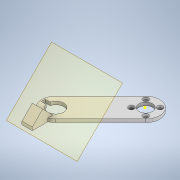
# Autodesk Inventor part: Pièce_moteur_maintient_test_6
Saved by Autodesk Inventor 2020.1 (Build 241239000, 239)
## iProperties
Created: 2019-07-26
Part Number: Pièce_moteur_maintient_test_6
Material: Générique
Document SubType Name: Modeling
Designer: marlo
Density: 1 g/cm^3
Appearance: Par défaut
Author: marlo
Autodesk Inventor part; units mm, degrees
ref_plane "YZ Plane" through (0, 0, 0) normal (1, 0, 0) x (0, 1, 0)
ref_plane "XZ Plane" through (0, 0, 0) normal (0, 1, 0) x (-1, 0, 0)
ref_plane "XY Plane" through (0, 0, 0) normal (0, 0, 1) x (1, 0, 0)
sketch "Esquisse3" plane through (0, 0, 0) normal (0, 1, 0) x (-1, 0, 0)
  line L0 (-7.087, 5.913) -> (5.913, 5.913) construction
  line L1 (5.913, 5.913) -> (5.913, -7.087) construction
  line L2 (5.913, -7.087) -> (-7.087, -7.087) construction
  line L3 (-7.087, -7.087) -> (-7.087, 5.913) construction
  line L4 (-7.087, 5.913) -> (5.913, -7.087) construction
  line L5 (5.913, 5.913) -> (-7.087, -7.087) construction
  line L6 (-12.087, 10.913) -> (10.913, 10.913) construction
  line L7 (10.913, 10.913) -> (10.913, -12.087) construction
  line L8 (10.913, -12.087) -> (-12.087, -12.087) construction
  line L9 (-12.087, -12.087) -> (-12.087, 10.913) construction
  line L10 (-12.087, 10.913) -> (10.913, -12.087) construction
  line L11 (10.913, 10.913) -> (-12.087, -12.087) construction
  line L12 (-7.087, 5.913) -> (-12.087, 5.913) construction
  line L13 (-12.087, 5.913) -> (-12.087, 10.913) construction
  line L14 (-12.087, 10.913) -> (-7.087, 10.913) construction
  line L15 (-7.087, 10.913) -> (-7.087, 5.913) construction
  line L16 (-7.087, -7.087) -> (-12.087, -7.087) construction
  line L17 (-12.087, -7.087) -> (-12.087, -12.087) construction
  line L18 (-12.087, -12.087) -> (-7.087, -12.087) construction
  line L19 (-7.087, -12.087) -> (-7.087, -7.087) construction
  line L20 (5.913, -7.087) -> (10.913, -7.087) construction
  line L21 (10.913, -7.087) -> (10.913, -12.087) construction
  line L22 (10.913, -12.087) -> (5.913, -12.087) construction
  line L23 (5.913, -12.087) -> (5.913, -7.087) construction
  line L24 (10.913, 10.913) -> (5.913, 10.913) construction
  line L25 (5.913, 10.913) -> (5.913, 5.913) construction
  line L26 (5.913, 5.913) -> (10.913, 5.913) construction
  line L27 (10.913, 5.913) -> (10.913, 10.913) construction
  circle A0 centre (8.413, 8.413) radius 2.5
  circle A1 centre (8.413, -9.587) radius 2.5
  circle A2 centre (-9.587, -9.587) radius 2.5
  circle A3 centre (-9.587, 8.413) radius 2.5
  circle A4 centre (-0.587, -0.587) radius 17.5
  circle A5 centre (-0.587, -0.587) radius 8.5
  circle A6 centre (55.9815, 55.9815) radius 17.5
  circle A7 centre (55.9815, 55.9815) radius 10
  line L28 (57.4815, 65.8684) -> (54.4815, 65.8684)
  line L29 (54.4815, 65.8684) -> (54.4815, 86.8684)
  line L30 (54.4815, 86.8684) -> (57.4815, 86.8684)
  line L31 (57.4815, 86.8684) -> (57.4815, 65.8684)
  line L32 (49.4815, 91.8684) -> (49.4815, 60.8684)
  line L33 (49.4815, 60.8684) -> (62.4815, 60.8684)
  line L34 (62.4815, 60.8684) -> (62.4815, 91.8684)
  line L35 (62.4815, 91.8684) -> (49.4815, 91.8684)
  line L36 (71.664, 53.4815) -> (65.664, 53.4815)
  line L37 (65.664, 53.4815) -> (65.664, 58.4815)
  line L38 (65.664, 58.4815) -> (71.664, 58.4815)
  line L39 (71.664, 58.4815) -> (71.664, 53.4815)
  line L40 (11.7873, -12.9614) -> (-12.9614, 11.7873) construction
  line L41 (11.7873, -12.9614) -> (68.3559, 43.6071)
  line L42 (-12.9614, 11.7873) -> (43.6071, 68.3559)
  line L43 (-12.9614, -12.9614) -> (68.3559, 68.3559) construction
  point P0 (-0.587, -0.587)
  point P1 (8.413, 8.413)
  point P2 (73.4815, 55.9815)
  point P3 (17.4356, 66.5)
  point P4 (62.4815, 72.2296)
  point P5 (49.4815, 72.2296)
  point P6 (57.4815, 73.4171)
  point P7 (54.4815, 73.4171)
  point P8 (49.4815, 63.5808)
  point P9 (62.4815, 63.5808)
  dimension "d1" = 13
  dimension "d2" = 13
  dimension "d3" = 5
  dimension "d4" = 35
  dimension "d9" = 9
  dimension "d31" = 35
  dimension "d32" = 20
  dimension "d33" = 3
  dimension "d34" = 21
  dimension "d36" = 5
  dimension "d37" = 5
  dimension "d51" = 6
  dimension "d56" = 115
  constraints: 88 end point, 20 parallel, 12 tangent, 11 point on circle, 9 perpendicular, 8 centre point, 8 horizontal, 6 coincident, 4 collinear, 2 midpoint, 2 point on line, 3 other
  measures "d1" distance of L0.end L1.end
  measures "d2" distance of L0.start L0.end
  measures "d3" distance between parallel lines of L2 L8
  measures "d4" diameter of A4
  measures "d9" radial gap between concentric circles of A4 A5
  measures "d31" diameter of A6
  measures "d32" diameter of A7
  measures "d33" distance of L29.end L30.end
  measures "d34" distance of L30.end L28.start
  measures "d36" distance between parallel lines of L29 L32
  measures "d37" distance of L38.end L36.start
  measures "d51" distance of L36.start L36.end
  measures "d56" distance of L43.start L43.end
extrude "Extrusion1" add sketch "Esquisse3" along normal blind 4 contours A4 | A4 L42 A6 L41 | A6 L32 A7 L36 L39 L38 L34 | L32 L35 L34 A6 L31 L30 L29 | A6 L29 A7 L32 | L34 A7 L31 A6
chamfer "Chanfrein5" distance 1 distance2 2 1 edges at (12.087, 4, -9.587) measured on face at (12.587, 4, -9.587)
chamfer "Chanfrein6" distance 1 distance2 2 1 edges at (-5.913, 4, -9.587) measured on face at (-5.413, 4, -9.587)
chamfer "Chanfrein7" distance 1 distance2 2 1 edges at (-5.913, 4, 8.413) measured on face at (-5.413, 4, 8.413)
chamfer "Chanfrein8" distance 1 distance2 2 1 edges at (12.087, 4, 8.413) measured on face at (12.587, 4, 8.413)
ref_plane "Plan de construction1" through (-62.4815, 4, 91.8684) normal (0, 0.7071068, 0.7071068) x (1, 0, 0)
sketch "Esquisse8" plane through (-62.4815, 4, 91.8684) normal (0, 0.7071068, 0.7071068) x (1, 0, 0)
  line L0 (0, 11.0583) -> (0, -2.8284) projected
  line L1 (0, 0) -> (13, 0)
  line L2 (13, 0) -> (13, 18.3465)
  line L3 (13, 18.3465) -> (0, 18.3465)
  line L4 (0, 18.3465) -> (0, 0)
  line L5 (8, 3.5355) -> (5, 3.5355) projected
  line L6 (8, 3.5355) -> (5, 3.5355)
  line L7 (5, 3.5355) -> (5, 18.3465)
  line L8 (5, 18.3465) -> (8, 18.3465)
  line L9 (8, 18.3465) -> (8, 3.5355)
  point P0 (62.4815, 62.1323)
  point P1 (8, 18.3465)
  constraints: 16 end point, 4 parallel, 2 horizontal, 2 perpendicular, 2 point on line
extrude "Extrusion3" add sketch "Esquisse8" against normal up to surface contours L4 L3 L7 L5 L9 L2 L1 L0 surface through (0.587, 4, -0.587) normal (0, 1, 0)
sketch "Esquisse9" plane through (-54.4815, 6.5, 89.3684) normal (0, 0.7071068, -0.7071068) x (-1, 0, 0)
  line L0 (0, -3.5355) -> (3, -3.5355) projected
  line L1 (0, -3.5355) -> (3, -3.5355)
  line L2 (3, -3.5355) -> (3, 0)
  line L3 (3, 0) -> (0, 0)
  line L4 (0, 0) -> (0, -3.5355)
  point P0 (-54.4815, -67.7892)
  constraints: 8 end point, 2 parallel, 1 horizontal, 1 perpendicular
extrude "Extrusion4" add sketch "Esquisse9" along normal up to surface (14.811 mm away)
sketch "Esquisse10" plane through (0, 4, 0) normal (0, 1, 0) x (1, 0, 0)
  point P0 (0, 0)
